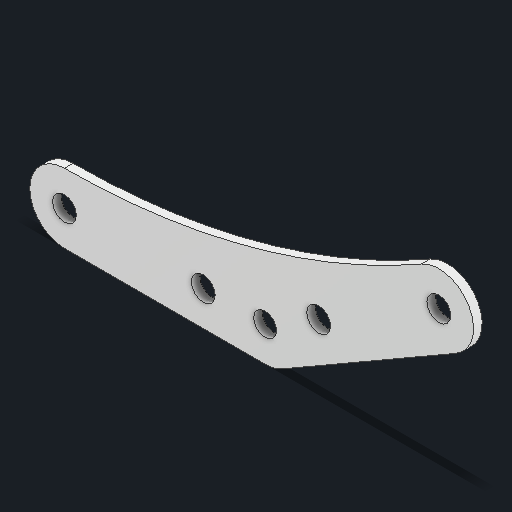
# Autodesk Inventor part: 60 Degree Gusset
Saved by Autodesk Inventor 2025.1 (Build 291241000, 241)
## iProperties
Created: 2024-10-22
Part Number: 60 Degree Gusset
Material: Acetal Resin, White
Document SubType Name: Modeling
Designer: averey
Density: 1.425 g/cm^3
Appearance: Smooth - White
Author: averey
Autodesk Inventor part; units mm, degrees
ref_plane "YZ Plane" through (0, 0, 0) normal (1, 0, 0) x (0, 1, 0)
ref_plane "XZ Plane" through (0, 0, 0) normal (0, 1, 0) x (-1, 0, 0)
ref_plane "XY Plane" through (0, 0, 0) normal (0, 0, 1) x (1, 0, 0)
sketch "main" plane through (0, 0, 0) normal (0, 0, 1) x (1, 0, 0)
  circle A0 centre (-6.1105, -12.0036) radius 2.1844
  circle A1 centre (-31.5105, -12.0036) radius 2.1844
  circle A2 centre (15.0202, -6.3416) radius 2.1844
  circle A3 centre (37.0172, 6.3584) radius 2.1844
  arc A4 (-31.5236, -5.6536) -> (-31.5105, -18.3536) centre (-31.5105, -12.0036) ccw
  arc A5 (40.1922, 0.8591) -> (33.8536, 11.8642) centre (37.0172, 6.3584) ccw
  arc A6 (-31.5236, -5.6536) -> (33.8536, 11.8642) centre (-31.796, 126.1175) ccw
  line L0 (-31.5105, -18.3536) -> (5.2134, -18.3536)
  line L1 (40.1922, 0.8591) -> (8.3884, -17.5028)
  circle A7 centre (5.2134, -12.0036) radius 2.0955
  arc A8 (5.2134, -18.3536) -> (8.3884, -17.5028) centre (5.2134, -12.0036) ccw
  line L2 (5.2134, -12.0036) -> (43.3134, -12.0036) construction
  point P0 (-0.7926, -1.6009)
  dimension "d0" = 12.7
  dimension "d3" = 12.7
  dimension "d7" = 4.191
  dimension "d8" = 6.35
  dimension "d13" = 25.4
  measures "d0" diameter of A4
  measures "d3" diameter of A5
  measures "d7" diameter of A7
  measures "d8" radius of A8
  measures "d13" distance of A3.centre A2.centre
sketch "Sketch1" plane through (0, 0, 0) normal (0, 0, 1) x (1, 0, 0)
  circle A0 centre (25.4, 0) radius 2.1844
  circle A1 centre (0, 0) radius 2.1844
  circle A2 centre (46.5307, 5.662) radius 2.1844
  circle A3 centre (68.5277, 18.362) radius 2.1844
  arc A4 (-0.0131, 6.35) -> (0, -6.35) centre (0, 0) ccw
  arc A5 (71.7027, 12.8627) -> (65.3641, 23.8678) centre (68.5277, 18.362) ccw
  arc A6 (-0.0131, 6.35) -> (65.3641, 23.8678) centre (-0.2855, 138.1211) ccw
  line L0 (0, -6.35) -> (36.7239, -6.35)
  line L1 (71.7027, 12.8627) -> (39.8989, -5.4993)
  circle A7 centre (36.7239, 0) radius 2.0955
  arc A8 (36.7239, -6.35) -> (39.8989, -5.4993) centre (36.7239, 0) ccw
  line L2 (36.7239, 0) -> (74.8239, 0) construction
  constraints: 1 other
extrude "Extrusion1" add sketch "Sketch1" along normal blind 1.5875
body "Solid1"
